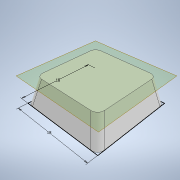
# Autodesk Inventor part: bottom
Saved by Autodesk Inventor 2022 (Build 260153000, 153)
## iProperties
Created: 2022-03-01
Part Number: bottom
Material: Generic
Document SubType Name: Modeling
Designer: Nathan Griffith
Density: 1 g/cm^3
Appearance: Default
Author: Nathan Griffith
Autodesk Inventor part; units mm, degrees
ref_plane "YZ Plane" through (0, 0, 0) normal (1, 0, 0) x (0, 1, 0)
ref_plane "XZ Plane" through (0, 0, 0) normal (0, 1, 0) x (-1, 0, 0)
sketch "Sketch1" plane through (0, 0, 0) normal (0, 1, 0) x (-1, 0, 0)
  line L0 (0, 0) -> (18, 0)
  line L1 (18, 0) -> (18, 18)
  line L2 (18, 18) -> (0, 18)
  line L3 (0, 18) -> (0, 0)
  dimension "d0" = 18
  dimension "d1" = 18
  constraints: 8 end point, 2 parallel, 1 horizontal, 1 perpendicular
  measures "d0" distance of L2.end L1.end
  measures "d1" distance of L1.end L0.end
extrude "Extrusion1" add sketch "Sketch1" along normal blind 8 draft -15
fillet "Fillet1" radius 1.5 8 edges at (-1.0718, 4, 16.9282) (-9, 8, 15.8564) (-2.1436, 8, 9) (-9, 8, 2.1436) (-1.0718, 4, 1.0718) (-16.9282, 4, 1.0718) (-16.9282, 4, 16.9282) (-15.8564, 8, 9)
ref_plane "Work Plane1" through (-9, 33.5885, 16.5511) normal (1, 0, 0) x (0, 0, -1)
sketch "Sketch2" plane through (-9, 33.5885, 16.5511) normal (1, 0, 0) x (0, 0, -1)
  line L0 (13.2565, -25.5885) -> (1.8457, -25.5885) projected
  arc A0 (14.7054, -26.7002) -> (13.2565, -25.5885) centre (13.2565, -27.0885) ccw projected
  arc A1 (1.8457, -25.5885) -> (13.2565, -25.5885) centre (7.5511, -8.5166) ccw
  point P0 (16.5511, -33.5885)
  point P1 (13.2565, -25.5885)
  dimension "d5" = 18
  constraints: 3 point on circle, 1 centre point
  measures "d5" radius of A1
extrude "Extrusion2" cut sketch "Sketch2" along normal through all both and the other way through all
sketch "Sketch3" plane through (0, 0, 0) normal (0, -1, 0) x (1, 0, 0)
  line L0 (-16.5511, 18) -> (-1.4489, 18) construction
  line L1 (-9, 18) -> (-9, 0) construction
  line L2 (-1.4489, 0) -> (-16.5511, 0) construction
  line L3 (-18, 1.4489) -> (-18, 16.5511) construction
  line L4 (-18, 9) -> (0, 9) construction
  line L5 (-1, 1) -> (-17, 1)
  line L6 (-17, 1) -> (-17, 17)
  line L7 (-17, 17) -> (-1, 17)
  line L8 (-1, 17) -> (-1, 1)
  line L9 (-1, 1) -> (-17, 17) construction
  line L10 (-17, 1) -> (-1, 17) construction
  point P0 (0, 0)
  point P1 (-9, 9)
  point P2 (-9, 9)
  dimension "d8" = 16
  dimension "d9" = 16
  constraints: 16 end point, 8 midpoint, 2 horizontal, 2 parallel, 1 perpendicular
  measures "d8" distance of L6.end L7.end
  measures "d9" distance of L7.end L5.start
extrude "Extrusion3" cut sketch "Sketch3" against normal blind 4.5 draft -15
sketch "Sketch4" plane through (0, 4.5, 0) normal (0, -1, 0) x (1, 0, 0)
  line L0 (-15.7942, 15.7942) -> (-15.7942, 2.2058) construction
  line L1 (-15.7942, 9) -> (-2.2058, 9) construction
  line L2 (-2.2058, 2.2058) -> (-2.2058, 15.7942) construction
  line L3 (-2.2058, 15.7942) -> (-15.7942, 15.7942) construction
  line L4 (-9, 15.7942) -> (-9, 2.2058) construction
  line L5 (-15.7942, 2.2058) -> (-2.2058, 2.2058) construction
  circle A0 centre (-9, 9) radius 2.775
  point P0 (0, 0)
  dimension "d12" = 5.55
  constraints: 5 midpoint, 4 end point, 1 centre point
  measures "d12" diameter of A0
extrude "Extrusion4" add sketch "Sketch4" along normal blind 4
sketch "Sketch5" plane through (-9, 0.5, 9) normal (0, -1, 0) x (1, 0, 0)
  line L0 (0.6, 2.075) -> (-0.6, 2.075)
  line L1 (-0.6, -2.075) -> (0.6, -2.075)
  line L2 (-0.6, 2.075) -> (0.6, -2.075) construction
  line L3 (-2.075, 0.6) -> (-2.075, -0.6)
  line L4 (2.075, -0.6) -> (2.075, 0.6)
  line L5 (2.075, 0.6) -> (-2.075, -0.6) construction
  line L6 (-2.075, 0.6) -> (2.075, -0.6) construction
  line L7 (-6.7942, 6.7942) -> (-6.7942, -6.7942) construction
  line L8 (-6.7942, 0) -> (6.7942, 0) construction
  line L9 (6.7942, -6.7942) -> (6.7942, 6.7942) construction
  line L10 (-6.7942, -6.7942) -> (6.7942, -6.7942) construction
  line L11 (0, -6.7942) -> (0, 6.7942) construction
  arc A0 (0.9, -0.6) -> (0.6, -0.9) centre (0.9, -0.9) ccw
  arc A1 (-0.6, -0.9) -> (-0.9, -0.6) centre (-0.9, -0.9) ccw
  arc A2 (0.6, 0.9) -> (0.9, 0.6) centre (0.9, 0.9) ccw
  arc A3 (-0.9, 0.6) -> (-0.6, 0.9) centre (-0.9, 0.9) ccw
  line L12 (-0.6, 2.075) -> (-0.6, 0.9)
  line L13 (-0.6, -0.9) -> (-0.6, -2.075)
  line L14 (-2.075, -0.6) -> (-0.9, -0.6)
  line L15 (-0.9, 0.6) -> (-2.075, 0.6)
  line L16 (0.6, 2.075) -> (0.1735, 0.6) construction
  line L17 (0, 0) -> (-0.6, -2.075) construction
  line L18 (2.075, 0.6) -> (0.9, 0.6)
  line L19 (0.9, -0.6) -> (2.075, -0.6)
  line L20 (0.6, -2.075) -> (0.6, -0.9)
  line L21 (0.6, 0.9) -> (0.6, 2.075)
  point P0 (9, -9)
  dimension "d15" = 1.2
  dimension "d16" = 4.15
  dimension "d17" = 4.15
  dimension "d18" = 1.2
  dimension "d19" = 0.3
  constraints: 38 end point, 10 parallel, 9 midpoint, 9 symmetric about line, 8 point on circle, 4 centre point, 4 perpendicular, 4 tangent, 3 horizontal, 1 vertical, 3 other
  measures "d15" distance of L1.end L1.start
  measures "d16" distance of L1.start L0.end
  measures "d17" distance of L4.start L3.end
  measures "d18" distance of L3.end L3.start
  measures "d19" radius of A0
extrude "Extrusion5" cut sketch "Sketch5" against normal blind 4
ref_plane "Work Plane3" through (0, 6, 0) normal (0, -1, 0) x (1, 0, 0)
split_face "Split1"
sketch "Sketch7" plane through (0, 6, 0) normal (0, -1, 0) x (1, 0, 0)
  line L0 (-25.6931, 27.6788) -> (12.1363, 27.6788)
  line L1 (12.1363, 27.6788) -> (12.1363, -37.3947)
  line L2 (12.1363, -37.3947) -> (-25.6931, -37.3947)
  line L3 (-25.6931, -37.3947) -> (-25.6931, 27.6788)
  point P0 (0, 0)
  constraints: 8 end point, 2 parallel, 1 horizontal, 1 perpendicular
extrude "Extrusion7" cut sketch "Sketch7" against normal blind 10
body "Solid1"
